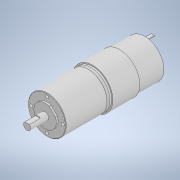
# Autodesk Inventor part: RS-775GM104 v1
Saved by Autodesk Inventor 2021 (Build 250183000, 183)
## iProperties
Created: 2022-01-31
Part Number: RS-775GM104 v1
Material: 一般
Document SubType Name: Modeling
Designer: hirohumi
Density: 1 g/cm^3
Appearance: 既定
Author: hirohumi
Autodesk Inventor part; units mm, degrees
ref_plane "YZ Plane" through (0, 0, 0) normal (1, 0, 0) x (0, 1, 0)
ref_plane "XZ Plane" through (0, 0, 0) normal (0, 1, 0) x (-1, 0, 0)
ref_plane "XY Plane" through (0, 0, 0) normal (0, 0, 1) x (1, 0, 0)
sketch "スケッチ1" plane through (0, 0, 0) normal (0, 0, 1) x (1, 0, 0)
  circle A0 centre (0, 0) radius 21.2
  dimension "d0" = 42.4
  constraints: 1 centre point, 1 coincident
  measures "d0" diameter of A0
extrude "押し出し1" add sketch "スケッチ1" against normal blind 5
sketch "スケッチ2" plane through (0, 0, -5) normal (0, 0, -1) x (-1, 0, 0)
  circle A0 centre (0, 0) radius 22.5
  dimension "d3" = 45
  constraints: 1 centre point, 1 coincident
  measures "d3" diameter of A0
extrude "押し出し2" add sketch "スケッチ2" along normal blind 30
sketch "スケッチ3" plane through (0, 0, -35) normal (0, 0, -1) x (-1, 0, 0)
  circle A0 centre (0, 0) radius 21.2
  dimension "d6" = 42.4
  constraints: 1 centre point, 1 coincident
  measures "d6" diameter of A0
extrude "押し出し3" add sketch "スケッチ3" along normal blind 28
fillet "フィレット1" radius 3 1 edges at (-21.2, 0, 0)
sketch "スケッチ4" plane through (0, 0, -63) normal (0, 0, -1) x (-1, 0, 0)
  line L0 (-1.75, 18.5) -> (1.75, 18.5)
  line L1 (1.75, 18.5) -> (1.75, 17.5)
  line L2 (1.75, 17.5) -> (-1.75, 17.5)
  line L3 (-1.75, 17.5) -> (-1.75, 18.5)
  line L4 (-1.75, -17.5) -> (1.75, -17.5)
  line L5 (1.75, -17.5) -> (1.75, -18.5)
  line L6 (1.75, -18.5) -> (-1.75, -18.5)
  line L7 (-1.75, -18.5) -> (-1.75, -17.5)
  point P0 (0, 0)
  dimension "d10" = 3.5
  dimension "d11" = 1
  dimension "d12" = 3.5
  dimension "d13" = 1
  dimension "d14" = 17.5
  dimension "d15" = 17.5
  dimension "d16" = 1.75
  constraints: 16 end point, 4 parallel, 2 horizontal, 2 perpendicular, 1 vertical alignment
  measures "d10" distance of L1.end L2.end
  measures "d11" distance of L0.end L1.end
  measures "d12" distance of L5.end L6.end
  measures "d13" distance of L4.end L5.end
  measures "d14" distance from line of point (0, 0) L2
  measures "d15" distance from line of point (0, 0) L4
  measures "d16" distance from line of point (0, 0) L3
extrude "押し出し4" add sketch "スケッチ4" along normal blind 9
sketch "スケッチ5" plane through (0, 0, 0) normal (0, 0, 1) x (1, 0, 0)
  circle A0 centre (0, 0) radius 21
  dimension "d19" = 42
  constraints: 1 centre point, 1 coincident
  measures "d19" diameter of A0
extrude "押し出し5" add sketch "スケッチ5" along normal blind 45.9
chamfer "面取り1" distance 0.5 angle 45 1 edges at (-21, 0, 45.9)
sketch "スケッチ6" plane through (0, 0, 45.9) normal (0, 0, 1) x (1, 0, 0)
  arc A0 (4.6676, 11.5958) -> (-11.5958, -4.6676) centre (0, 0) ccw
  line L0 (4.6676, 11.5958) -> (11.5958, 4.6676)
  line L1 (-11.5958, -4.6676) -> (-4.6676, -11.5958)
  line L2 (11.5958, 4.6676) -> (9.2337, 4.6676) construction
  arc A1 (11.5958, 4.6676) -> (4.6676, 11.5958) centre (0, 0) ccw construction
  arc A2 (-11.5958, -4.6676) -> (-4.6676, -11.5958) centre (0, 0) ccw construction
  arc A3 (-4.6676, -11.5958) -> (11.5958, 4.6676) centre (0, 0) ccw
  dimension "d25" = 25
  dimension "d26" = 11.5
  dimension "d27" = 23
  dimension "d28" = 45
  constraints: 9 point on circle, 6 end point, 4 centre point, 1 coincident, 1 horizontal, 1 parallel
  measures "d25" diameter of A0
  measures "d26" distance from line of point (0, 0) L0
  measures "d27" distance between parallel lines of L0 L1
  measures "d28" angle of L2 L0
extrude "押し出し6" add sketch "スケッチ6" along normal blind 2
sketch "スケッチ7" plane through (0, 0, 47.9) normal (0, 0, 1) x (1, 0, 0)
  circle A0 centre (0, 0) radius 4
  dimension "d31" = 8
  constraints: 1 centre point, 1 coincident
  measures "d31" diameter of A0
extrude "押し出し7" add sketch "スケッチ7" along normal blind 20
sketch "スケッチ8" plane through (0, 0, 67.9) normal (0, 0, 1) x (1, 0, 0)
  circle A0 centre (0, 0) radius 4 projected
  arc A1 (-2.6458, 3) -> (2.6458, 3) centre (0, 0) ccw
  line L0 (-2.6458, 3) -> (2.6458, 3)
  point P0 (2.6458, 3)
  dimension "d34" = 3
  constraints: 2 end point, 2 point on circle, 1 centre point, 1 coincident, 1 horizontal, 2 other
  measures "d34" distance from line of point (0, 0) L0
extrude "押し出し8" cut sketch "スケッチ8" against normal blind 12 contours L0 A0 picked at (-0.6179, 3.1815)
sketch "スケッチ9" plane through (0, 0, 45.9) normal (0, 0, 1) x (1, 0, 0)
  circle A0 centre (0, 17.5) radius 1.75
  circle A1 centre (-17.5, 0) radius 1.75
  circle A2 centre (0, -17.5) radius 1.75
  circle A3 centre (17.5, 0) radius 1.75
  point P0 (0, 0)
  dimension "d37" = 3.5
  dimension "d38" = 17.5
  dimension "d41" = 360
  constraints: 4 centre point, 1 vertical alignment, 9 other
  measures "d37" diameter of A0
  measures "d38" distance of point (0, 0) A0.centre
extrude "押し出し9" cut sketch "スケッチ9" against normal blind 12
